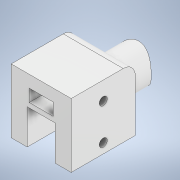
# Autodesk Inventor part: korob_3
Saved by Autodesk Inventor 2020 (Build 240168000, 168)
## iProperties
Created: 2019-12-25
Part Number: korob_3
Material: ABS Plastic
Document SubType Name: Modeling
Designer: metal
Density: 1.06 g/cm^3
Appearance: Smooth - White
Author: metal
Autodesk Inventor part; units mm, degrees
ref_plane "YZ Plane" through (0, 0, 0) normal (1, 0, 0) x (0, 1, 0)
ref_plane "XZ Plane" through (0, 0, 0) normal (0, 1, 0) x (-1, 0, 0)
ref_plane "XY Plane" through (0, 0, 0) normal (0, 0, 1) x (1, 0, 0)
sketch "Sketch1" plane through (0, 0, 0) normal (0, 0, 1) x (1, 0, 0)
  line L0 (0, 0) -> (15, 0)
  line L1 (15, 0) -> (15, -16)
  line L2 (15, -16) -> (0, -16)
  line L3 (0, -16) -> (0, 0)
  dimension "d0" = 16
  dimension "d1" = 15
  constraints: 8 end point, 2 parallel, 1 horizontal, 1 perpendicular
  measures "d0" distance of L2.end L0.start
  measures "d1" distance of L0.start L0.end
extrude "Extrusion1" add sketch "Sketch1" along normal blind 16
sketch "Sketch21" plane through (0, 0, 0) normal (0, 0, -1) x (-1, 0, 0)
  circle A0 centre (-7.5, -8) radius 4.5
  line L0 (0, 0) -> (0, -16) projected
  line L1 (-15, 0) -> (0, 0) projected
  dimension "d2" = 16
  dimension "d89" = 9
  dimension "d90" = 7.5
  dimension "d91" = 8
  constraints: 1 centre point
  measures "d89" diameter of A0
  measures "d90" distance from line of L0 A0.centre
  measures "d91" distance from line of L1 A0.centre
extrude "Extrusion12" add sketch "Sketch21" along normal blind 10
sketch "Sketch22" plane through (7.5, -8, -10) normal (0, 0, -1) x (-1, 0, 0)
  ellipse E0 centre (0, 0) end of major axis (0, -3) minor radius 1.8
  point P0 (7.5, 8)
  dimension "d2" = 16
  dimension "d94" = 1.8
  dimension "d95" = 3
  constraints: 2 other
extrude "Extrusion13" cut sketch "Sketch22" against normal blind 8
ref_plane "Work Plane5" through (7.5, -3.5, 0) normal (0, -1, 0) x (1, 0, 0)
sketch "Sketch24" plane through (7.5, -3.5, 0) normal (0, -1, 0) x (1, 0, 0)
  line L0 (-4.5, -10) -> (4.5, -10) projected
  line L1 (4.5, -10) -> (-4.5, -10)
  line L2 (-4.5, -10) -> (-4.5, -7)
  line L3 (-4.5, 0) -> (-4.5, -10) projected
  line L4 (4.5, -10) -> (4.5, -7)
  line L5 (4.5, 0) -> (4.5, -10) projected
  arc A0 (-4.5, -7) -> (4.5, -7) centre (0, -0.3856) ccw
  point P0 (-7.5, 0)
  dimension "d2" = 16
  dimension "d98" = 3
  dimension "d99" = 3
  dimension "d100" = 8
  constraints: 6 end point, 2 point on circle, 2 point on line, 1 centre point, 1 horizontal
  measures "d98" distance of L0.start L2.end
  measures "d99" distance of L0.end L4.end
  measures "d100" radius of A0
extrude "Extrusion14" cut sketch "Sketch24" along normal blind 12
sketch "Sketch31" plane through (0, 0, 16) normal (0, 0, 1) x (1, 0, 0)
  line L0 (4.5, -3) -> (10.5, -3)
  line L1 (10.5, -3) -> (10.5, -6.1)
  line L2 (10.5, -6.1) -> (4.5, -6.1)
  line L3 (4.5, -6.1) -> (4.5, -3)
  line L4 (15, -16) -> (15, 0) projected
  line L5 (15, 0) -> (0, 0) projected
  dimension "d2" = 16
  dimension "d130" = 3.1
  dimension "d131" = 6
  dimension "d132" = 4.5
  dimension "d133" = 3
  constraints: 8 end point, 2 parallel, 1 horizontal, 1 perpendicular
  measures "d130" distance of L0.end L1.end
  measures "d131" distance of L0.start L0.end
  measures "d132" distance between parallel lines of L4 L1
  measures "d133" distance between parallel lines of L5 L0
extrude "Extrusion20" cut sketch "Sketch31" against normal blind 6
sketch "Sketch32" plane through (0, 0, 16) normal (0, 0, 1) x (1, 0, 0)
  line L0 (4, -7.284) -> (11, -7.284)
  line L1 (11, -7.284) -> (11, -16.284)
  line L2 (11, -16.284) -> (4, -16.284)
  line L3 (4, -16.284) -> (4, -7.284)
  line L4 (10.5, -6.1) -> (4.5, -6.1) projected
  line L5 (15, -16) -> (15, 0) projected
  point P0 (0, 0)
  dimension "d2" = 16
  dimension "d140" = 7
  dimension "d141" = 1.184
  dimension "d142" = 4
  dimension "d143" = 9
  constraints: 8 end point, 2 parallel, 1 horizontal, 1 perpendicular
  measures "d140" distance of L0.start L0.end
  measures "d141" distance between parallel lines of L4 L0
  measures "d142" distance between parallel lines of L5 L1
  measures "d143" distance of L2.end L0.start
extrude "Extrusion21" cut sketch "Sketch32" against normal blind 15
sketch "Sketch33" plane through (0, -16, 0) normal (-1, 0, 0) x (0, 0, 1)
  circle A0 centre (8, 11.45) radius 1
  line L0 (16, 0) -> (16, 16) projected
  point P0 (0, 16)
  dimension "d2" = 16
  dimension "d146" = 2
  dimension "d147" = 8
  dimension "d148" = 4.55
  constraints: 1 centre point
  measures "d146" diameter of A0
  measures "d147" distance from line of L0 A0.centre
  measures "d148" vertical distance of point (0, 16) A0.centre
extrude "Extrusion22" cut sketch "Sketch33" against normal through all
sketch "Sketch34" plane through (0, 0, 0) normal (0, 0, -1) x (-1, 0, 0)
  line L0 (0, -16) -> (-15, -16) projected
  line L1 (-11, -16) -> (-4, -16)
  line L2 (-4, -16) -> (-4, -12.9958)
  line L3 (-4, -12.9958) -> (-11, -12.9958)
  line L4 (-11, -12.9958) -> (-11, -16)
  line L5 (0, 0) -> (0, -16) projected
  dimension "d2" = 16
  dimension "d151" = 7
  dimension "d152" = 4
  constraints: 8 end point, 2 parallel, 1 horizontal, 1 perpendicular, 1 point on line
  measures "d151" distance of L2.end L3.end
  measures "d152" distance between parallel lines of L5 L2
extrude "Extrusion23" cut sketch "Sketch34" against normal blind 10
sketch "Sketch35" plane through (15, -16, 0) normal (1, 0, 0) x (0, 0, -1)
  circle A0 centre (-8, 2.45) radius 1
  line L0 (0, 0) -> (-16, 0) projected
  line L1 (-16, 0) -> (-16, 16) projected
  point P0 (0, 16)
  dimension "d2" = 16
  dimension "d155" = 2
  dimension "d156" = 2.45
  dimension "d157" = 8
  constraints: 1 centre point
  measures "d155" diameter of A0
  measures "d156" distance from line of L0 A0.centre
  measures "d157" distance from line of L1 A0.centre
extrude "Extrusion24" cut sketch "Sketch35" against normal through all
fillet "Fillet4" radius 3 1 edges at (7.5, 0, 0)
body "Solid1"
